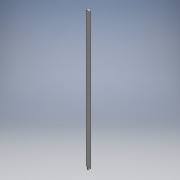
# Autodesk Inventor part: brade
Saved by Autodesk Inventor 2016 SP1 (Build 200210100, 210)
## iProperties
Created: 2017-01-17
Part Number: brade
Material: 一般
Document SubType Name: Modeling
Designer: p_admin
Density: 1 g/cm^3
Appearance: 既定
Author: p_admin
Autodesk Inventor part; units mm, degrees
ref_plane "YZ Plane" through (0, 0, 0) normal (1, 0, 0) x (0, 1, 0)
ref_plane "XZ Plane" through (0, 0, 0) normal (0, 1, 0) x (-1, 0, 0)
ref_plane "XY Plane" through (0, 0, 0) normal (0, 0, 1) x (1, 0, 0)
sketch "スケッチ1" plane through (0, 0, 0) normal (0, 0, 1) x (1, 0, 0)
  line L0 (0, 0) -> (0, 10)
  line L1 (0, 10) -> (17.3205, 0)
  line L2 (0, 10) -> (20, 10) construction
  line L3 (0, 0) -> (17.3205, 0)
  dimension "d0" = 20
  dimension "d1" = 30
  dimension "d2" = 10
  constraints: 8 end point, 1 equal length, 1 horizontal, 1 vertical
  measures "d0" distance of L0.end L1.end
  measures "d1" angle of L1 L2
  measures "d2" distance of L0.start L0.end
extrude "押し出し1" add sketch "スケッチ1" along normal blind 40
sketch "スケッチ2" plane through (0, 0, 0) normal (0, 0, -1) x (-1, 0, 0)
  circle A0 centre (-3.5, 3.5) radius 3
  line L0 (0, 10) -> (0, 0) projected
  line L1 (0, 0) -> (-6.3397, 6.3397)
  line L2 (-17.3205, 0) -> (0, 10) projected
  line L3 (0, 0) -> (8.9658, 0) construction
  line L4 (-17.3205, 0) -> (0, 0) projected
  dimension "d5" = 6
  dimension "d6" = 135
  dimension "d7" = 0
  dimension "d8" = 3.5
  constraints: 4 end point, 1 centre point, 1 equal length, 1 horizontal, 1 point on line
  measures "d5" diameter of A0
  measures "d6" angle of L3 L1
  measures "d7" distance from line of L1 A0.centre
  measures "d8" distance from line of L4 A0.centre
extrude "押し出し2" add sketch "スケッチ2" along normal blind 10 contours A0 L1 | L1 A0
shell "シェル1" thickness 1 removed faces 1 at (2.3486, 4.7468, -10)
sketch "スケッチ3" plane through (0, 0, 0) normal (0, -1, 0) x (1, 0, 0)
  circle A0 centre (3.2619, -5) radius 1.6
  line L0 (0.5, -10) -> (6.5, -10) projected
  point P0 (0, 0)
  dimension "d12" = 3.2
  dimension "d13" = 5
  constraints: 1 centre point
  measures "d12" diameter of A0
  measures "d13" distance from line of L0 A0.centre
extrude "押し出し3" cut sketch "スケッチ3" against normal blind 7.5
sketch "スケッチ4" plane through (3.5, 3.5, -10) normal (0, 0, -1) x (-1, 0, 0)
  circle A0 centre (0, 0) radius 3
  point P0 (3.5, -3.5)
  constraints: 1 centre point
extrude "押し出し4" cut sketch "スケッチ4" against normal blind 8
sketch "スケッチ5" plane through (3.5, 3.5, -2) normal (0, 0, -1) x (-1, 0, 0)
  circle A0 centre (0, 0) radius 2
  circle A1 centre (0, 0) radius 3
  circle A2 centre (0, 0) radius 3 projected
  line L0 (0.0001, -3) -> (0.0001, -2.7)
  line L1 (0.0001, -2.7) -> (-1.3077, -2.7)
  line L2 (0.0001, -2.7) -> (1.3079, -2.7) construction
  line L3 (-1.3077, -2.7) -> (1.3077, -2.7)
  point P0 (3.5, -3.5)
  dimension "d18" = 0.3
  dimension "d19" = 180
  dimension "d20" = 0
  constraints: 8 end point, 3 point on circle, 1 centre point, 1 coincident, 1 collinear, 1 horizontal, 1 vertical, 3 other
  measures "d18" distance of L0.start L0.end
  measures "d19" angle of L1 L2
  measures "d20" distance between parallel lines of L3 L1
extrude "押し出し5" add sketch "スケッチ5" along normal blind 8 contours A1 L3 L1
sketch "スケッチ6" plane through (2.1923, 0.8, -2) normal (0, -1, 0) x (1, 0, 0)
  circle A0 centre (1.3, -4) radius 1.1
  line L0 (2.6153, -8) -> (0, -8) projected
  line L1 (0, 0) -> (0, -8) projected
  point P0 (-2.1923, 2)
  dimension "d23" = 2.2
  dimension "d24" = 4
  dimension "d25" = 1.3
  constraints: 1 centre point
  measures "d23" diameter of A0
  measures "d24" distance from line of L0 A0.centre
  measures "d25" distance from line of A0.centre L1
extrude "押し出し6" cut sketch "スケッチ6" against normal blind 8
sketch "スケッチ7" plane through (3.5, 3.5, -10) normal (0, 0, -1) x (-1, 0, 0)
  circle A0 centre (0, 0) radius 3.1532
  point P0 (3.5, -3.5)
  constraints: 1 centre point
extrude "押し出し7" cut sketch "スケッチ7" against normal blind 0.5
sketch "スケッチ8" plane through (0, 0, 40) normal (0, 0, 1) x (1, 0, 0)
  line L0 (0, 0) -> (0, 10) projected
  line L1 (0, 10) -> (17.3205, 0) projected
  line L2 (0, 0) -> (0, 10)
  line L3 (0, 10) -> (17.3205, 0)
  line L4 (17.3205, 0) -> (0, 0)
  constraints: 6 end point, 1 perpendicular, 1 vertical
extrude "押し出し8" add sketch "スケッチ8" along normal blind 460
shell "シェル2" thickness 1 removed faces 1 at (5.1962, 3.4226, 39)
